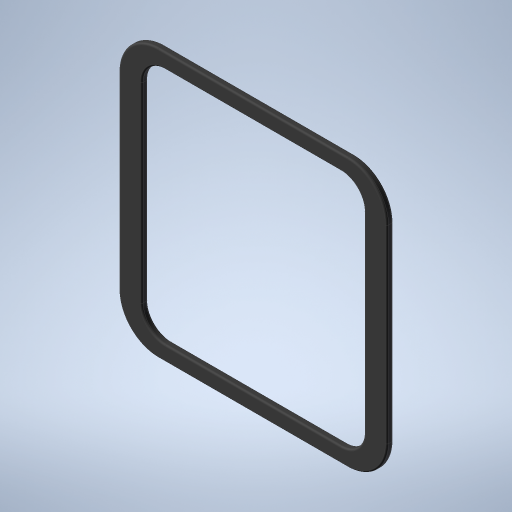
# Autodesk Inventor part: LeptonBlockSpacer
Saved by Autodesk Inventor 2023 (Build 270158000, 158)
## iProperties
Created: 2025-12-12
Part Number: LeptonBlockSpacer
Material: Generic
Document SubType Name: Modeling
Designer: DanAr
Density: 1 g/cm^3
Appearance: Default
Author: DanAr
Autodesk Inventor part; units mm, degrees
ref_plane "YZ Plane" through (0, 0, 0) normal (1, 0, 0) x (0, 1, 0)
ref_plane "XZ Plane" through (0, 0, 0) normal (0, 1, 0) x (-1, 0, 0)
ref_plane "XY Plane" through (0, 0, 0) normal (0, 0, 1) x (1, 0, 0)
sketch "Sketch1" plane through (0, 0, 0) normal (0, 0, 1) x (1, 0, 0)
  line L0 (0, 0) -> (28.2, 0)
  line L1 (28.2, 0) -> (28.2, 30.2)
  line L2 (28.2, 30.2) -> (0, 30.2)
  line L3 (0, 30.2) -> (0, 0)
  line L4 (14.1, 30.2) -> (14.1, 0)
  line L5 (31.1, -1.9) -> (-2.9, -1.9)
  line L6 (-2.9, -1.9) -> (-2.9, 32.1)
  line L7 (-2.9, 32.1) -> (31.1, 32.1)
  line L8 (31.1, 32.1) -> (31.1, -1.9)
  line L9 (31.1, -1.9) -> (-2.9, 32.1) construction
  line L10 (-2.9, -1.9) -> (31.1, 32.1) construction
  point P0 (14.1, 15.1)
  dimension "d0" = 30.2
  dimension "d1" = 28.2
  dimension "d2" = 34
  dimension "d3" = 34
  constraints: 22 end point, 5 midpoint, 4 parallel, 2 horizontal, 2 perpendicular
  measures "d0" distance of L0.end L1.end
  measures "d1" distance of L1.end L2.end
  measures "d2" distance of L6.end L7.end
  measures "d3" distance of L7.end L5.start
extrude "Extrusion1" add sketch "Sketch1" along normal blind 0.8
fillet "Fillet1" radius 3 4 edges at (0, 0, 0.4) (0, 30.2, 0.4) (28.2, 30.2, 0.4) (28.2, 0, 0.4)
fillet "Fillet2" radius 5 4 edges at (31.1, 32.1, 0.4) (-2.9, 32.1, 0.4) (31.1, -1.9, 0.4) (-2.9, -1.9, 0.4)
fillet "Fillet3" radius 0.2 24 edges at (-1.4355, 30.6355, 0) (-2.9, 15.1, 0) (-1.4355, -0.4355, 0) (14.1, -1.9, 0) (29.6355, -0.4355, 0) (31.1, 15.1, 0) (29.6355, 30.6355, 0) (14.1, 32.1, 0) (14.1, 32.1, 0.8) (29.6355, 30.6355, 0.8) (31.1, 15.1, 0.8) (29.6355, -0.4355, 0.8) (14.1, -1.9, 0.8) (-1.4355, -0.4355, 0.8) (-2.9, 15.1, 0.8) (-1.4355, 30.6355, 0.8) (0, 15.1, 0.8) (14.1, 0, 0.8) (28.2, 15.1, 0.8) (14.1, 30.2, 0.8) (14.1, 30.2, 0) (28.2, 15.1, 0) (14.1, 0, 0) (0, 15.1, 0)
body "Solid1"
